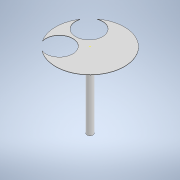
# Autodesk Inventor part: rack holder
Saved by Autodesk Inventor 2021.3 (Build 253353010, 353A)
## iProperties
Created: 2021-07-06
Part Number: rack holder
Material: Generic
Document SubType Name: Modeling
Designer: Dell
Density: 1 g/cm^3
Appearance: Default
Author: Dell
Autodesk Inventor part; units mm, degrees
ref_plane "YZ Plane" through (0, 0, 0) normal (1, 0, 0) x (0, 1, 0)
ref_plane "XZ Plane" through (0, 0, 0) normal (0, 1, 0) x (-1, 0, 0)
ref_plane "XY Plane" through (0, 0, 0) normal (0, 0, 1) x (1, 0, 0)
sketch "Sketch1" plane through (0, 0, 0) normal (0, 1, 0) x (-1, 0, 0)
  circle A0 centre (0, 0) radius 113.0198
  arc A1 (67.1662, 90.8965) -> (94.7779, 61.5681) centre (52.1094, 49.0592) ccw
  arc A2 (94.7779, -61.5681) -> (67.1662, -90.8965) centre (52.195, -49.1397) ccw
  constraints: 8 point on circle, 3 centre point, 1 coincident
extrude "Extrusion1" add sketch "Sketch1" along normal blind 1 contours A0 A2 A1
sketch "Sketch3" plane through (0, 0, 0) normal (0, -1, 0) x (1, 0, 0)
  point P0 (0, 0)
sketch "Sketch7" plane through (0, 0, 0) normal (0, -1, 0) x (1, 0, 0)
  circle A0 centre (0, 0) radius 9.8515
  constraints: 1 centre point, 1 coincident
extrude "Extrusion3" add sketch "Sketch7" along normal blind 246.38
body "Solid1"
